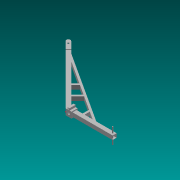
# Autodesk Inventor part: kepala baru
Saved by Autodesk Inventor 2014 SP2 (Build 180246200, 246)
## iProperties
Created: 2019-07-15
Part Number: kepala baru
Material: Steel, Mild
Document SubType Name: Modeling
Designer: USER PC
Density: 7.86 g/cm^3
Appearance: Steel
Author: USER PC
Autodesk Inventor part; units mm, degrees
ref_plane "YZ Plane" through (0, 0, 0) normal (1, 0, 0) x (0, 1, 0)
ref_plane "XZ Plane" through (0, 0, 0) normal (0, 1, 0) x (-1, 0, 0)
ref_plane "XY Plane" through (0, 0, 0) normal (0, 0, 1) x (1, 0, 0)
sketch "Sketch1" plane through (0, 0, 0) normal (0, 0, 1) x (1, 0, 0)
  line L0 (0, 0) -> (150, 0)
  line L1 (150, 0) -> (150, 150)
  line L2 (150, 150) -> (0, 150)
  line L3 (0, 150) -> (0, 0)
  line L4 (0, 0) -> (-1500, 1500)
  line L5 (-1500, 1500) -> (-1429.2893, 1570.7107)
  line L6 (-1429.2893, 1570.7107) -> (0, 141.4214)
  line L7 (0, 141.4214) -> (0, 0)
  line L8 (150, 100) -> (150, 0)
  line L9 (150, 0) -> (150, 125)
  line L10 (150, 125) -> (850, 125)
  line L11 (850, 125) -> (850, 25)
  line L12 (850, 25) -> (150, 25)
  line L13 (150, 25) -> (150, 125)
  dimension "d0" = 150
  dimension "d1" = 150
  dimension "d8" = 1500
  dimension "d9" = 100
  dimension "d12" = 125
  dimension "d13" = 700
  dimension "d14" = 100
  constraints: 28 end point, 5 perpendicular, 4 parallel, 1 collinear, 1 horizontal, 1 point on line
  measures "d0" distance of L2.end L1.end
  measures "d1" distance of L1.end L0.end
  measures "d8" horizontal distance of L0.start L4.end
  measures "d9" distance of L4.end L5.end
  measures "d12" distance of L0.end L9.end
  measures "d13" distance of L9.end L10.end
  measures "d14" distance of L10.end L11.end
extrude "Extrusion3" add sketch "Sketch1" along normal mid plane 150 contours L3 L2 L1 L0
sketch "Sketch3" plane through (0, 0, 0) normal (0, 0, 1) x (1, 0, 0)
  line L0 (0, 0) -> (-1500, 1500)
  line L1 (0, 0) -> (2121.3203, 0) construction
  line L2 (-1500, 1500) -> (-1429.2893, 1570.7107)
  line L3 (-1429.2893, 1570.7107) -> (0, 141.4214)
  line L4 (0, 0) -> (0, 141.4214)
  line L5 (150, 0) -> (150, 125)
  line L6 (150, 125) -> (850, 125)
  line L7 (850, 125) -> (850, 25)
  line L8 (850, 25) -> (150, 25)
  line L9 (150, 25) -> (150, 125)
  dimension "d17" = 135
  dimension "d18" = 1500
  dimension "d19" = 100
  dimension "d20" = 125
  dimension "d21" = 700
  dimension "d22" = 100
  constraints: 20 end point, 5 perpendicular, 3 parallel, 1 equal length, 1 horizontal, 1 point on line
  measures "d17" angle of L1 L0
  measures "d18" horizontal distance of L0.start L0.end
  measures "d19" distance of L0.end L2.end
  measures "d20" distance of L5.start L5.end
  measures "d21" distance of L5.end L6.end
  measures "d22" distance of L6.end L7.end
extrude "Extrusion4" add sketch "Sketch3" along normal mid plane 100
sketch "Sketch4" plane through (-1500, 1500, -50) normal (-0.7071068, 0.7071068, 0) x (-0.7071068, -0.7071068, 0)
  line L0 (-95.5, 95.5) -> (-4.5, 95.5)
  line L1 (-4.5, 95.5) -> (-4.5, 4.5)
  line L2 (-4.5, 4.5) -> (-95.5, 4.5)
  line L3 (-95.5, 4.5) -> (-95.5, 95.5)
  line L4 (-95.5, 95.5) -> (-4.5, 4.5) construction
  line L5 (-4.5, 95.5) -> (-95.5, 4.5) construction
  line L6 (0, 100) -> (0, 0) projected
  line L7 (-100, 100) -> (0, 100) projected
  point P0 (0, 50)
  point P1 (-50, 50)
  dimension "d25" = 91
  dimension "d26" = 91
  dimension "d102" = 4.5
  dimension "d103" = 4.5
  constraints: 12 end point, 2 midpoint, 2 parallel, 1 horizontal, 1 perpendicular
  measures "d25" distance of L1.end L2.end
  measures "d26" distance of L0.end L1.end
  measures "d102" distance between parallel lines of L0 L7
  measures "d103" distance between parallel lines of L6 L1
extrude "Extrusion5" cut sketch "Sketch4" against normal blind 2122.5
sketch "Sketch5" plane through (0, 0, 0) normal (0, 0, 1) x (1, 0, 0)
  line L0 (0, 132.8216) -> (69.0672, 132.8216)
  line L1 (69.0672, 132.8216) -> (69.0672, 2.6564)
  line L2 (69.0672, 2.6564) -> (0, 2.6564)
  line L3 (0, 2.6564) -> (0, 132.8216)
  point P0 (0, 0)
  constraints: 8 end point, 2 parallel, 1 horizontal, 1 perpendicular
extrude "Extrusion6" add sketch "Sketch5" along normal mid plane 100.5
sketch "Sketch6" plane through (0, 0, 0) normal (0, 0, 1) x (1, 0, 0)
  point P0 (0, 0)
sketch "Sketch7" plane through (0, 150, 75) normal (0, 1, 0) x (1, 0, 0)
  circle A0 centre (75, 75) radius 30
  point P0 (0, 75)
  dimension "d31" = 60
  constraints: 1 centre point
  measures "d31" diameter of A0
extrude "Extrusion7" cut sketch "Sketch7" against normal blind 340
sketch "Sketch8" plane through (850, 25, 50) normal (1, 0, 0) x (0, 0, -1)
  line L0 (4.5, 95.5) -> (95.5, 95.5)
  line L1 (95.5, 95.5) -> (95.5, 4.5)
  line L2 (95.5, 4.5) -> (4.5, 4.5)
  line L3 (4.5, 4.5) -> (4.5, 95.5)
  line L4 (4.5, 95.5) -> (95.5, 4.5) construction
  line L5 (95.5, 95.5) -> (4.5, 4.5) construction
  line L6 (0, 100) -> (100, 100) projected
  line L7 (100, 100) -> (100, 0) projected
  point P0 (50, -25)
  point P1 (50, 50)
  dimension "d34" = 91
  dimension "d35" = 91
  dimension "d104" = 4.5
  dimension "d105" = 4.5
  constraints: 12 end point, 2 midpoint, 2 parallel, 1 horizontal, 1 perpendicular
  measures "d34" distance of L1.end L2.end
  measures "d35" distance of L0.end L1.end
  measures "d104" distance between parallel lines of L0 L6
  measures "d105" distance between parallel lines of L7 L1
extrude "Extrusion8" cut sketch "Sketch8" against normal blind 700
sketch "Sketch9" plane through (0, 0, 0) normal (0, 0, 1) x (1, 0, 0)
  point P0 (0, 0)
sketch "Sketch10" plane through (0, 0, 0) normal (0, 0, 1) x (1, 0, 0)
  line L0 (150, 125) -> (550, 125)
  line L1 (550, 125) -> (-971.9923, 1113.3934)
  line L2 (550, 125) -> (2376.4621, 125) construction
  line L3 (550, 125) -> (641.8039, 125)
  line L4 (641.8039, 125) -> (-1142.0421, 1283.4431)
  line L5 (-971.9923, 1113.3934) -> (-1142.0421, 1283.4431)
  line L6 (-971.9923, 1113.3934) -> (-731.5056, 1113.3934) construction
  line L7 (150, 125) -> (300, 125)
  point P0 (0, 0)
  dimension "d41" = 147
  dimension "d42" = 50
  dimension "d43" = 400
  dimension "d44" = 135
  dimension "d45" = 150
  constraints: 16 end point, 3 horizontal, 2 point on line, 1 equal length, 1 parallel
  measures "d41" angle of L2 L1
  measures "d42" distance between parallel lines of L4 L1
  measures "d43" distance of L0.start L0.end
  measures "d44" angle of L6 L5
  measures "d45" distance of L0.start L7.end
extrude "Extrusion9" add sketch "Sketch10" along normal mid plane 100
sketch "Sketch11" plane through (0, 0, 50) normal (0, 0, 1) x (1, 0, 0)
  line L0 (850, 125) -> (641.8039, 125) projected
  line L1 (641.8039, 125) -> (-1141.9842, 1283.4055) projected
  line L2 (-1141.9842, 1283.4055) -> (-1429.2893, 1570.7107) projected
  line L3 (-1429.2893, 1570.7107) -> (-1500, 1500) projected
  line L4 (-1500, 1500) -> (0, 0) projected
  line L5 (0, 141.4214) -> (0, 0) projected
  line L6 (0, 141.4214) -> (-971.9344, 1113.3558) projected
  line L7 (-971.9344, 1113.3558) -> (550, 125) projected
  line L8 (550, 125) -> (150, 125) projected
  line L9 (150, 25) -> (150, 125) projected
  line L10 (150, 25) -> (850, 25) projected
  line L11 (850, 25) -> (850, 125) projected
  line L12 (150, 125) -> (300, 125)
  line L13 (300, 125) -> (300, 287.3519)
  line L14 (300, 125) -> (350, 125)
  line L15 (350, 125) -> (350, 254.8815)
  line L16 (300, 287.3519) -> (350, 254.8815)
  line L17 (305, 130) -> (305, 278.143)
  line L18 (0, 141.4214) -> (-212.132, 353.5534)
  line L19 (-212.132, 353.5534) -> (-50.6311, 515.0544)
  line L20 (-212.132, 353.5534) -> (-247.4874, 388.9087)
  line L21 (-247.4874, 388.9087) -> (-93.5014, 542.8947)
  line L22 (-93.5014, 542.8947) -> (-50.6311, 515.0544)
  line L23 (0, 141.4214) -> (-459.6194, 601.0408)
  line L24 (-459.6194, 601.0408) -> (-350.7235, 709.9367)
  line L25 (-459.6194, 601.0408) -> (-494.9747, 636.3961)
  line L26 (-494.9747, 636.3961) -> (-393.5938, 737.777)
  line L27 (-350.7235, 709.9367) -> (-393.5938, 737.777)
  dimension "d48" = 150
  dimension "d49" = 50
  dimension "d51" = 300
  dimension "d52" = 50
  dimension "d54" = 650
  dimension "d55" = 50
  constraints: 32 end point, 11 point on line, 6 perpendicular, 2 collinear, 1 midpoint
  measures "d48" distance of L8.end L12.end
  measures "d49" distance of L12.end L14.end
  measures "d51" distance of L5.start L18.end
  measures "d52" distance of L18.end L20.end
  measures "d54" distance of L5.start L23.end
  measures "d55" distance of L23.end L25.end
sketch "Sketch12" plane through (0, 141.4214, -50) normal (0.7071068, 0.7071068, 0) x (-0.7071068, 0.7071068, 0)
  line L0 (0, 100) -> (1374.5228, 100) projected
  line L1 (1374.5228, 0) -> (0, 0) projected
  line L2 (0, 100) -> (300, 100)
  line L3 (300, 100) -> (300, 0)
  line L4 (300, 0) -> (350, 0)
  line L5 (350, 0) -> (350, 100)
  line L6 (300, 100) -> (350, 100)
  line L7 (345, 95) -> (345, 5)
  line L8 (345, 5) -> (305, 5)
  line L9 (305, 5) -> (305, 95)
  line L10 (305, 95) -> (345, 95)
  line L11 (0, 100) -> (650, 100)
  line L12 (650, 100) -> (650, 0)
  line L13 (650, 0) -> (700, 0)
  line L14 (700, 0) -> (700, 100)
  line L15 (650, 100) -> (700, 100)
  line L16 (695, 95) -> (695, 5)
  line L17 (695, 5) -> (655, 5)
  line L18 (655, 5) -> (655, 95)
  line L19 (655, 95) -> (695, 95)
  point P0 (-100, 50)
  dimension "d56" = 300
  dimension "d57" = 50
  dimension "d58" = 5
  dimension "d59" = 650
  dimension "d60" = 50
  dimension "d61" = 5
  constraints: 36 end point, 8 point on line, 6 perpendicular, 1 collinear, 6 other
  measures "d56" distance of L0.start L2.end
  measures "d57" distance of L3.end L4.end
  measures "d58" distance between parallel lines of L5 L7
  measures "d59" distance of L0.start L11.end
  measures "d60" distance of L12.end L13.end
  measures "d61" distance between parallel lines of L14 L16
extrude "Extrusion10" add sketch "Sketch12" along normal blind 228.5 contours L0 L5 L1 L3 | L0 L14 L1 L12
sketch "Sketch13" plane through (0, 0, 50) normal (0, 0, 1) x (1, 0, 0)
  line L0 (-314.5783, 746.0819) -> (-298.0455, 762.6147) projected
  line L1 (-333.4008, 797.97) -> (-298.0455, 762.6147) projected
  line L2 (-357.4486, 773.9222) -> (-333.4008, 797.97) projected
  line L3 (-971.9344, 1113.3558) -> (-393.5938, 737.777) projected
  line L4 (-314.5783, 746.0819) -> (-357.4486, 773.9222)
  line L5 (-333.4008, 797.97) -> (-298.0455, 762.6147)
  line L6 (-298.0455, 762.6147) -> (-314.5783, 746.0819)
  line L7 (-333.4008, 797.97) -> (-357.4486, 773.9222)
  constraints: 8 end point, 1 collinear, 1 parallel, 1 perpendicular, 1 point on line
extrude "Extrusion11" cut sketch "Sketch13" against normal blind 228.5
sketch "Sketch15" plane through (150, 125, 50) normal (0, 1, 0) x (1, 0, 0)
  line L0 (0, 100) -> (400, 100) projected
  line L1 (400, 0) -> (0, 0) projected
  line L2 (0, 0) -> (150, 0)
  line L3 (150, 0) -> (150, 100)
  line L4 (150, 100) -> (200, 100)
  line L5 (200, 100) -> (200, 0)
  line L6 (150, 0) -> (200, 0)
  line L7 (195, 5) -> (195, 95)
  line L8 (195, 95) -> (155, 95)
  line L9 (155, 95) -> (155, 5)
  line L10 (155, 5) -> (195, 5)
  point P0 (-150, 50)
  dimension "d66" = 150
  dimension "d67" = 50
  dimension "d68" = 5
  constraints: 18 end point, 2 midpoint, 2 point on line, 1 collinear, 1 perpendicular, 3 other
  measures "d66" distance of L1.end L2.end
  measures "d67" distance of L3.end L4.end
  measures "d68" distance between parallel lines of L5 L7
extrude "Extrusion12" add sketch "Sketch15" along normal blind 163.5
sketch "Sketch16" plane through (0, 0, 0) normal (0, 0, 1) x (1, 0, 0)
  point P0 (0, 0)
sketch "Sketch17" plane through (-1429.2893, 1570.7107, -50) normal (0.7071068, 0.7071068, 0) x (-0.7071068, 0.7071068, 0)
  line L0 (0, 0) -> (-406.3108, 0) projected
  line L1 (-406.3108, 100) -> (0, 100) projected
  line L2 (0, 100) -> (0, 115)
  line L3 (0, 115) -> (-300, 115)
  line L4 (-300, -15) -> (0, -15)
  line L5 (0, -15) -> (0, 0)
  line L6 (0, 100) -> (-250, 100)
  line L7 (-7.859, 0) -> (-250, 0)
  line L8 (-300, 115) -> (-300, 100)
  line L9 (-300, 0) -> (-300, -15)
  line L10 (-300, 100) -> (-250, 100)
  line L11 (-300, 0) -> (-250, 0)
  point P0 (-2121.3203, 50)
  dimension "d71" = 15
  dimension "d72" = 15
  dimension "d74" = 300
  constraints: 20 end point, 5 perpendicular, 5 point on line, 3 collinear, 1 parallel
  measures "d71" distance of L1.end L2.end
  measures "d72" distance of L4.end L0.start
  measures "d74" distance of L4.start L4.end
extrude "Extrusion17" add sketch "Sketch17" against normal blind 100
sketch "Sketch22" plane through (-1141.9842, 1283.4055, -50) normal (0.7071068, 0.7071068, 0) x (-0.7071068, 0.7071068, 0)
  line L0 (406.3108, 115) -> (406.3108, -15) projected
  line L1 (406.3108, 0) -> (206.3108, 0)
  line L2 (206.3108, 0) -> (206.3108, 100)
  line L3 (206.3108, 100) -> (406.3108, 100)
  line L4 (406.3108, 100) -> (406.3108, 0)
  point P0 (-1715.0095, 50)
  dimension "d93" = 200
  constraints: 8 end point, 2 parallel, 1 horizontal, 1 perpendicular, 1 point on line
  measures "d93" distance of L2.end L3.end
extrude "Extrusion18" cut sketch "Sketch22" against normal blind 100
sketch "Sketch23" plane through (-1217.1573, 1358.5786, -65) normal (0, 0, -1) x (-0.7071068, -0.7071068, 0)
  line L0 (0, 0) -> (100, 0) projected
  line L1 (0, 300) -> (100, 300) projected
  line L2 (50, 110) -> (50, 180)
  circle A0 centre (50, 180) radius 20
  point P0 (100, -1821.3203)
  dimension "d96" = 70
  dimension "d97" = 110
  dimension "d98" = 40
  constraints: 2 end point, 1 centre point, 1 coincident, 1 perpendicular
  measures "d96" distance of L2.start L2.end
  measures "d97" distance from line of L0 L2.start
  measures "d98" diameter of A0
extrude "Extrusion19" cut sketch "Sketch23" against normal blind 433.5
fillet "Fillet2" radius 50 4 edges at (-1429.2893, 1570.7107, 57.5) (-1429.2893, 1570.7107, -57.5) (-1500, 1500, -57.5) (-1500, 1500, 57.5)
sketch "Sketch24" plane through (0, 0, 0) normal (0, 0, 1) x (1, 0, 0)
  line L0 (150, 125) -> (550, 125)
  line L1 (550, 125) -> (-971.9923, 1113.3934)
  line L2 (550, 125) -> (2376.4621, 125) construction
  line L3 (550, 125) -> (641.8039, 125)
  line L4 (641.8039, 125) -> (-1142.0421, 1283.4431)
  line L5 (-971.9923, 1113.3934) -> (-1142.0421, 1283.4431)
  line L6 (-971.9923, 1113.3934) -> (-731.5056, 1113.3934) construction
  line L7 (150, 125) -> (300, 125)
  line L8 (-1108.5856, 1256.3506) -> (-969.1448, 1116.9098)
  line L9 (551.333, 129.5) -> (-969.5414, 1117.1674)
  line L10 (626.6122, 129.5) -> (-1108.5856, 1256.3506)
  line L11 (551.333, 129.5) -> (626.6122, 129.5)
  line L12 (551.333, 129.5) -> (626.6122, 129.5)
  line L13 (626.6122, 129.5) -> (-1108.5856, 1256.3506)
  line L14 (-1108.5856, 1256.3506) -> (-969.1448, 1116.9098)
  line L15 (-969.1448, 1116.9098) -> (551.333, 129.5)
  point P0 (0, 0)
  point P1 (0, 0)
  dimension "d106" = 147
  dimension "d107" = 50
  dimension "d108" = 400
  dimension "d109" = 135
  dimension "d110" = 150
  dimension "d111" = 4.5
  dimension "d112" = 4.5
  dimension "d113" = 4.5
  dimension "d114" = 4.5
  constraints: 32 end point, 4 collinear, 3 horizontal, 3 parallel, 2 point on line, 1 equal length
  measures "d106" angle of L2 L1
  measures "d107" distance between parallel lines of L4 L1
  measures "d108" distance of L0.start L0.end
  measures "d109" angle of L6 L5
  measures "d110" distance of L0.start L7.end
  measures "d111" distance between parallel lines of L10 L4
  measures "d112" distance between parallel lines of L1 L9
  measures "d113" distance between parallel lines of L3 L11
  measures "d114" distance between parallel lines of L8 L5
extrude "Extrusion20" cut sketch "Sketch24" along normal mid plane 91 contours L10 L11 L9 L8
sketch "Sketch26" plane through (0, 0, 0) normal (0, 0, 1) x (1, 0, 0)
  point P0 (0, 0)
sketch "Sketch27" plane through (850, 25, 50) normal (1, 0, 0) x (0, 0, -1)
  line L0 (0, 100) -> (100, 100) projected
  line L1 (0, 0) -> (0, 100) projected
  line L2 (0, 0) -> (100, 0) projected
  line L3 (100, 100) -> (100, 0) projected
  line L4 (4.5, 95.5) -> (100, 95.5)
  line L5 (100, 95.5) -> (100, 0)
  line L6 (100, 0) -> (4.5, 0)
  line L7 (4.5, 0) -> (4.5, 95.5)
  line L8 (4.5, 95.5) -> (95.5, 95.5)
  line L9 (95.5, 95.5) -> (95.5, 4.5)
  line L10 (95.5, 4.5) -> (4.5, 4.5)
  line L11 (4.5, 4.5) -> (4.5, 95.5)
  point P0 (50, -25)
  constraints: 16 end point, 4 parallel, 2 horizontal, 2 perpendicular
extrude "Extrusion21" add sketch "Sketch27" along normal blind 300 contours L0 L3 L4 L7 L2 L1 | L3 L2 L7 L10 L9 L4
sketch "Sketch28" plane through (0, 0, 50) normal (0, 0, 1) x (1, 0, 0)
  line L0 (1150, 125) -> (1150, 25) projected
  line L1 (641.8039, 125) -> (1150, 125) projected
  circle A0 centre (1100, 75) radius 10
  dimension "d120" = 50
  dimension "d121" = 50
  dimension "d122" = 20
  constraints: 1 centre point
  measures "d120" distance from line of L0 A0.centre
  measures "d121" distance from line of A0.centre L1
  measures "d122" diameter of A0
extrude "Extrusion22" add sketch "Sketch28" along normal blind 150 and the other way blind 250
sketch "Sketch29" plane through (0, 0, 75) normal (0, 0, 1) x (1, 0, 0)
  line L0 (0, 0) -> (150, 0) projected
  line L1 (150, 0) -> (150, 150) projected
  line L2 (150, 150) -> (0, 150) projected
  line L3 (50, 150) -> (100, 150)
  line L4 (100, 150) -> (100, 0)
  line L5 (100, 0) -> (50, 0)
  line L6 (50, 0) -> (50, 150)
  dimension "d127" = 50
  dimension "d128" = 50
  constraints: 8 end point, 2 parallel, 2 point on line, 1 horizontal, 1 perpendicular
  measures "d127" distance of L4.end L5.end
  measures "d128" distance between parallel lines of L1 L4
extrude "Extrusion23" add sketch "Sketch29" along normal blind 50 contours L6 L2 L4 L0
sketch "Sketch30" plane through (0, 150, -75) normal (0, 1, 0) x (1, 0, 0)
  circle A0 centre (75, -175) radius 15
  point P0 (0, -75)
  dimension "d131" = 30
  constraints: 1 centre point
  measures "d131" diameter of A0
extrude "Extrusion24" cut sketch "Sketch30" against normal blind 281
body "Solid1"
